Autodesk Inventor part; units mm, degrees
(part 2 of 2)
  point P20 (-50.834886, 12.533639)
  point P21 (-50.854476, 12.562862)
  point P22 (-101.999257, 156.659446)
  point P23 (-106.89852, 174.341704)
  point P24 (-50.834886, 12.533639)
  point P25 (-50.854476, 12.562862)
  point P26 (-101.999257, 156.659446)
  point P27 (-106.89852, 174.341704)
  point P28 (-50.834886, 12.533639)
  point P29 (-50.854476, 12.562862)
  point P30 (-101.999257, 156.659446)
  point P31 (-106.89852, 174.341704)
  point P32 (-50.834886, 12.533639)
  point P33 (-50.854476, 12.562862)
  constraints: 16 end point, 13 point on circle, 6 centre point, 2 point on line, 131 other
extrude "Extrusion2" cut sketch "Sketch3" along normal blind 8.382 contours L6 A1 E24 E23 A7 L11 L1 | L1 L11 A6 L6 | A1 L7 A8 A7 E23 E24
sketch "Sketch4" plane through (204.446927, 89.953752, 21.5392) normal (0, 0, 1) x (-0.622646, 0.7825036, 0)
  line L0 (-3.192917, 163.875478) -> (-3.192917, 2.602537)
  arc A0 (-3.192917, 163.875478) -> (-9.611038, 191.201711) centre (-64.575, 163.875478) ccw
  line L1 (-10.954295, 193.903537) -> (-9.611038, 191.201711)
  arc A1 (-6.678359, 192.474597) -> (-10.954295, 193.903537) centre (-9.525, 191.068446) ccw
  arc A2 (0, 163.875478) -> (-6.678359, 192.474597) centre (-64.575, 163.875478) ccw
  line L2 (0, 0) -> (0, 163.875478)
  arc A3 (0, 0) -> (-3.192917, 2.602537) centre (-29.65, -33.116159) ccw
  point P0 (56.90893, 215.989808)
extrude "Extrusion3" cut sketch "Sketch4" against normal blind 8.382
sketch "Sketch5" plane through (204.446927, 89.953752, 43.0784) normal (0, 0, 1) x (-0.622646, 0.7825036, 0)
  arc A0 (-6.678359, 192.474597) -> (-12.7, 191.068446) centre (-9.525, 191.068446) ccw
  line L0 (-12.7, 191.068446) -> (-12.7, 7.975202)
  arc A1 (0, 0) -> (-12.7, 7.975202) centre (-29.65, -33.116159) ccw
  line L1 (0, 0) -> (0, 163.875478)
  arc A2 (0, 163.875478) -> (-6.678359, 192.474597) centre (-64.575, 163.875478) ccw
  arc A3 (0, 0) -> (-12.7, 7.975202) centre (-29.65, -33.116159) ccw
  line L2 (-12.7, 7.975202) -> (0, 7.975202) construction
  line L3 (0, 0) -> (0, 163.875478)
  line L4 (-6.35, 7.975202) -> (-6.35, 163.875478)
  circle A4 centre (-6.35, 163.875478) radius 2.413
  circle A5 centre (-6.35, 113.075478) radius 2.413
  circle A6 centre (-6.35, 62.275478) radius 2.413
  circle A7 centre (-6.35, 11.475478) radius 2.413
  point P0 (56.90893, 215.989808)
  dimension "d11" = 4.826
  dimension "d14" = 50.8
  constraints: 4 centre point, 4 coincident, 4 end point, 2 vertical, 1 midpoint, 1 perpendicular, 1 point on line, 9 other
  measures "d11" diameter of A4
  measures "d14" distance of A4.centre A5.centre
ref_plane "Work Plane4" through (-228.588234, -244.583471, 0) normal (0, 0, 1) x (1, 0, 0)
extrude "Extrusion4" cut sketch "Sketch5" against normal up to surface (43.0784 mm away) contours A7 L4 | L4 A7 | A6 L4 | L4 A6 | A5 L4 | L4 A5 | A4
thread "Thread1" size "10-24 UNC" class "2B" standard "ANSI Unified Screw Threads" full length
thread "Thread2" size "10-24 UNC" class "2B" standard "ANSI Unified Screw Threads" full length
thread "Thread3" size "10-24 UNC" class "2B" standard "ANSI Unified Screw Threads" full length
thread "Thread4" size "10-24 UNC" class "2B" standard "ANSI Unified Screw Threads" full length
fillet "Fillet2" radius 3.175 2 edges at (204.4469, 89.9538, 36.4998) (206.1139, 75.0502, 21.5392)
sketch "Sketch6" plane through (76.213772, -12.082664, 43.0784) normal (-0.622646, 0.7825036, 0) x (0, 0, -1)
  line L0 (29.9212, 30.028059) -> (29.9212, 28.599119)
  line L1 (29.9212, 28.599119) -> (43.0784, 28.599119)
  line L2 (43.0784, 28.599119) -> (43.0784, 27.192968)
  line L3 (43.0784, 27.192968) -> (0, 27.192968)
  line L4 (0, 27.192968) -> (0, 28.599119)
  line L5 (0, 28.599119) -> (13.1572, 28.599119)
  line L6 (13.1572, 28.599119) -> (13.1572, 30.028059)
  line L7 (13.1572, 30.028059) -> (29.9212, 30.028059)
  line L8 (0, -157.403571) -> (0, -160.042775)
  line L9 (0, -160.042775) -> (43.0784, -160.042775)
  line L10 (43.0784, -160.042775) -> (43.0784, -157.403571)
  line L11 (43.0784, -157.403571) -> (29.9212, -157.403571)
  line L12 (29.9212, -157.403571) -> (29.9212, -160.57852)
  line L13 (29.9212, -160.57852) -> (13.1572, -160.57852)
  line L14 (13.1572, -160.57852) -> (13.1572, -157.403571)
  line L15 (13.1572, -157.403571) -> (0, -157.403571)
  line L16 (0, 27.192968) -> (0, 30.367968)
  line L17 (43.0784, -160.578569) -> (0, -160.578569)
  line L18 (0, -160.578569) -> (0, 30.367968)
  line L19 (0, 30.367968) -> (43.0784, 30.367968)
  line L20 (43.0784, 30.367968) -> (43.0784, -160.578569)
  point P0 (43.0784, 52.11433)
  constraints: 8 end point, 2 parallel, 1 horizontal, 1 perpendicular
sketch "Sketch7" plane through (62.84278, -38.952053, 0) normal (0.622646, -0.7825036, 0) x (0.7825036, 0.622646, 0)
  line L0 (-2.835091, 13.1572) -> (-1.406151, 13.1572)
  line L1 (-1.406151, 13.1572) -> (-1.406151, 0)
  line L2 (-1.406151, 0) -> (0, 0)
  line L3 (0, 0) -> (0, 43.0784)
  line L4 (-3.175, 43.0784) -> (-1.406151, 43.0784)
  line L5 (-1.406151, 43.0784) -> (-1.406151, 29.9212)
  line L6 (-1.406151, 29.9212) -> (-2.835091, 29.9212)
  line L7 (-2.835091, 29.9212) -> (-2.835091, 13.1572)
  line L8 (181.020673, 43.0784) -> (181.020673, 0)
  line L9 (0, 43.0784) -> (181.020673, 43.0784)
  line L10 (0, 0) -> (0, 43.0784)
  line L11 (0, 0) -> (181.020673, 0)
  line L12 (184.596538, 43.0784) -> (187.235743, 43.0784)
  line L13 (187.235743, 43.0784) -> (187.235743, 0)
  line L14 (187.235743, 0) -> (184.596538, 0)
  line L15 (184.596538, 0) -> (184.596538, 13.1572)
  line L16 (184.596538, 13.1572) -> (187.771488, 13.1572)
  line L17 (187.771488, 13.1572) -> (187.771488, 29.9212)
  line L18 (187.771488, 29.9212) -> (184.596538, 29.9212)
  line L19 (184.596538, 29.9212) -> (184.596538, 43.0784)
  line L20 (187.771538, 0) -> (184.596538, 0)
  line L21 (-3.175, 43.0784) -> (-3.175, 43.0784)
  line L22 (187.771538, 0) -> (-3.175, 0)
  line L23 (-3.175, 0) -> (-3.175, 43.0784)
  line L24 (-3.175, 43.0784) -> (187.771538, 43.0784)
  line L25 (187.771538, 43.0784) -> (187.771538, 0)
  point P0 (-24.921362, 0)
  constraints: 8 end point, 2 parallel, 1 horizontal, 1 perpendicular
ref_plane "Work Plane6" through (58.370314, -38.430454, 0) normal (0.7860048, 0.6182204, 0) x (-0.6182204, 0.7860048, 0)
ref_plane "Work Plane5" through (203.855103, 85.402445, 0) normal (0.7860048, 0.6182204, 0) x (-0.6182204, 0.7860048, 0)
sketch "Sketch8" plane through (116.421139, -62.612835, 43.0784) normal (0, 0, 1) x (0.784274, -0.6204146, 0)
  arc A0 (-15.535771, 161.593992) -> (-16.666713, 164.813097) centre (-18.627592, 162.315983) ccw
  arc A1 (-21.679175, 169.410851) -> (-16.666713, 164.813097) centre (10.785584, 199.7727) ccw
  arc A2 (-21.679175, 169.410851) -> (-27.089907, 167.964138) centre (-23.998086, 167.242147) ccw
  line L0 (-27.089907, 167.964138) -> (-62.88325, 14.684261)
  arc A3 (-62.88325, 14.684261) -> (-62.88325, -14.684261) centre (0, 0) ccw
  arc A4 (-62.88325, -14.684261) -> (-56.699609, -14.684261) centre (-59.791429, -13.962271) ccw
  line L1 (-56.699609, -14.684261) -> (-15.535771, 161.593992)
  circle A5 centre (-33.595916, 112.178541) radius 2.413
  circle A6 centre (-45.147762, 62.709411) radius 2.413
  circle A7 centre (-22.04407, 161.647671) radius 2.413
  circle A8 centre (-56.699609, 13.24028) radius 2.413
  line L2 (-23.276096, 170.333968) -> (-14.000634, 168.167997)
  line L3 (-14.000634, 168.167997) -> (-15.860711, 160.202484)
  arc A9 (-21.679175, 169.410851) -> (-27.089907, 167.964138) centre (-23.998086, 167.242147) ccw
  line L4 (-60.51342, -17.054091) -> (-57.421599, -17.776082)
  line L5 (-57.421599, -17.776082) -> (-56.699609, -14.684261)
  point P0 (-130.15199, -23.123759)
  point P1 (-15.535771, 161.593992)
  constraints: 8 end point, 2 collinear, 2 perpendicular, 2 point on circle, 2 tangent
extrude "Extrusion5" add sketch "Sketch8" against normal up to surface (43.0784 mm away) contours A0 A1 A2 L2 L3 | L5 L4 A4
body "Solid1"
